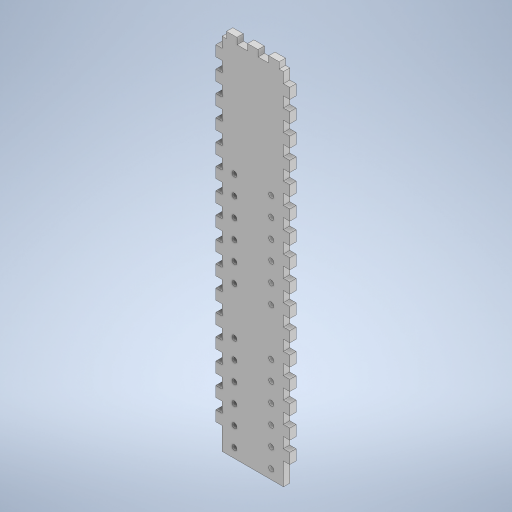
# Autodesk Inventor part: Module_supportX_MFC
Saved by Autodesk Inventor 2023 (Build 270158000, 158)
## iProperties
Created: 2022-11-01
Part Number: Module_supportX_MFC
Material: Generic
Document SubType Name: Modeling
Designer: incep
Density: 1 g/cm^3
Appearance: Default
Author: incep
Autodesk Inventor part; units mm, degrees
ref_plane "YZ Plane" through (0, 0, 0) normal (1, 0, 0) x (0, 1, 0)
ref_plane "XZ Plane" through (0, 0, 0) normal (0, 1, 0) x (-1, 0, 0)
ref_plane "XY Plane" through (0, 0, 0) normal (0, 0, 1) x (1, 0, 0)
sketch "Sketch1" plane through (0, 0, 0) normal (0, 0, 1) x (1, 0, 0)
  line L0 (29.075, 0) -> (29.075, -341.3) construction
  line L1 (29.075, -341.3) -> (-29.075, -341.3)
  line L2 (-29.075, -341.3) -> (-29.075, 0) construction
  line L3 (-5, 6) -> (5, 6)
  line L4 (5, 6) -> (5, 0)
  line L5 (-5, 0) -> (-5, 6)
  line L6 (-29.075, 0) -> (-5, 0) construction
  line L7 (5, 0) -> (29.075, 0) construction
  line L8 (15, 6) -> (25, 6)
  line L9 (25, 6) -> (25, 0)
  line L10 (15, 0) -> (15, 6)
  line L11 (-25, 6) -> (-15, 6)
  line L12 (-15, 6) -> (-15, 0)
  line L13 (-25, 0) -> (-25, 6)
  line L14 (-5, 6) -> (5, 6)
  line L15 (5, 6) -> (5, 0)
  line L16 (-5, 0) -> (-5, 6)
  line L17 (-29.075, 0) -> (-25, 0)
  line L18 (-15, 0) -> (-5, 0)
  line L19 (5, 0) -> (15, 0)
  line L20 (25, 0) -> (29.075, 0)
  line L21 (-35.075, -10) -> (-29.075, -10)
  line L22 (-29.075, -10) -> (-29.075, -20) construction
  line L23 (-29.075, -20) -> (-35.075, -20)
  line L24 (-35.075, -20) -> (-35.075, -10)
  line L25 (-29.075, -20) -> (-29.075, -30)
  line L26 (-29.075, 0) -> (-29.075, -10)
  line L27 (-35.075, -30) -> (-29.075, -30)
  line L28 (-29.075, -40) -> (-29.075, -50)
  line L29 (-29.075, -40) -> (-35.075, -40)
  line L30 (-35.075, -40) -> (-35.075, -30)
  line L31 (-35.075, -50) -> (-29.075, -50)
  line L32 (-29.075, -60) -> (-29.075, -70)
  line L33 (-29.075, -60) -> (-35.075, -60)
  line L34 (-35.075, -60) -> (-35.075, -50)
  line L35 (-35.075, -70) -> (-29.075, -70)
  line L36 (-29.075, -80) -> (-29.075, -90)
  line L37 (-29.075, -80) -> (-35.075, -80)
  line L38 (-35.075, -80) -> (-35.075, -70)
  line L39 (-35.075, -90) -> (-29.075, -90)
  line L40 (-29.075, -100) -> (-29.075, -110)
  line L41 (-29.075, -100) -> (-35.075, -100)
  line L42 (-35.075, -100) -> (-35.075, -90)
  line L43 (-35.075, -110) -> (-29.075, -110)
  line L44 (-29.075, -120) -> (-29.075, -130)
  line L45 (-29.075, -120) -> (-35.075, -120)
  line L46 (-35.075, -120) -> (-35.075, -110)
  line L47 (-35.075, -130) -> (-29.075, -130)
  line L48 (-29.075, -140) -> (-29.075, -150)
  line L49 (-29.075, -140) -> (-35.075, -140)
  line L50 (-35.075, -140) -> (-35.075, -130)
  line L51 (-35.075, -150) -> (-29.075, -150)
  line L52 (-29.075, -160) -> (-29.075, -170)
  line L53 (-29.075, -160) -> (-35.075, -160)
  line L54 (-35.075, -160) -> (-35.075, -150)
  line L55 (-35.075, -170) -> (-29.075, -170)
  line L56 (-29.075, -180) -> (-29.075, -190)
  line L57 (-29.075, -180) -> (-35.075, -180)
  line L58 (-35.075, -180) -> (-35.075, -170)
  line L59 (-35.075, -190) -> (-29.075, -190)
  line L60 (-29.075, -200) -> (-29.075, -210)
  line L61 (-29.075, -200) -> (-35.075, -200)
  line L62 (-35.075, -200) -> (-35.075, -190)
  line L63 (-35.075, -210) -> (-29.075, -210)
  line L64 (-29.075, -220) -> (-29.075, -230)
  line L65 (-29.075, -220) -> (-35.075, -220)
  line L66 (-35.075, -220) -> (-35.075, -210)
  line L67 (-35.075, -230) -> (-29.075, -230)
  line L68 (-29.075, -240) -> (-29.075, -250)
  line L69 (-29.075, -240) -> (-35.075, -240)
  line L70 (-35.075, -240) -> (-35.075, -230)
  line L71 (-35.075, -250) -> (-29.075, -250)
  line L72 (-29.075, -260) -> (-29.075, -270)
  line L73 (-29.075, -260) -> (-35.075, -260)
  line L74 (-35.075, -260) -> (-35.075, -250)
  line L75 (-35.075, -270) -> (-29.075, -270)
  line L76 (-29.075, -280) -> (-29.075, -290)
  line L77 (-29.075, -280) -> (-35.075, -280)
  line L78 (-35.075, -280) -> (-35.075, -270)
  line L79 (-35.075, -290) -> (-29.075, -290)
  line L80 (-29.075, -300) -> (-29.075, -310)
  line L81 (-29.075, -300) -> (-35.075, -300)
  line L82 (-35.075, -300) -> (-35.075, -290)
  line L83 (-35.075, -310) -> (-29.075, -310)
  line L84 (-29.075, -320) -> (-29.075, -330)
  line L85 (-29.075, -320) -> (-35.075, -320)
  line L86 (-35.075, -320) -> (-35.075, -310)
  line L87 (-29.075, -330) -> (-29.075, -341.3)
  line L88 (0, 0) -> (0, -341.3) construction
  line L89 (29.075, -341.3) -> (29.075, 0) construction
  line L90 (35.075, -10) -> (29.075, -10)
  line L91 (29.075, -10) -> (29.075, -20) construction
  line L92 (29.075, -20) -> (35.075, -20)
  line L93 (35.075, -20) -> (35.075, -10)
  line L94 (29.075, -20) -> (29.075, -30)
  line L95 (29.075, 0) -> (29.075, -10)
  line L96 (35.075, -30) -> (29.075, -30)
  line L97 (29.075, -40) -> (29.075, -50)
  line L98 (29.075, -40) -> (35.075, -40)
  line L99 (35.075, -40) -> (35.075, -30)
  line L100 (35.075, -50) -> (29.075, -50)
  line L101 (29.075, -60) -> (29.075, -70)
  line L102 (29.075, -60) -> (35.075, -60)
  line L103 (35.075, -60) -> (35.075, -50)
  line L104 (35.075, -70) -> (29.075, -70)
  line L105 (29.075, -80) -> (29.075, -90)
  line L106 (29.075, -80) -> (35.075, -80)
  line L107 (35.075, -80) -> (35.075, -70)
  line L108 (35.075, -90) -> (29.075, -90)
  line L109 (29.075, -100) -> (29.075, -110)
  line L110 (29.075, -100) -> (35.075, -100)
  line L111 (35.075, -100) -> (35.075, -90)
  line L112 (35.075, -110) -> (29.075, -110)
  line L113 (29.075, -120) -> (29.075, -130)
  line L114 (29.075, -120) -> (35.075, -120)
  line L115 (35.075, -120) -> (35.075, -110)
  line L116 (35.075, -130) -> (29.075, -130)
  line L117 (29.075, -140) -> (29.075, -150)
  line L118 (29.075, -140) -> (35.075, -140)
  line L119 (35.075, -140) -> (35.075, -130)
  line L120 (35.075, -150) -> (29.075, -150)
  line L121 (29.075, -160) -> (29.075, -170)
  line L122 (29.075, -160) -> (35.075, -160)
  line L123 (35.075, -160) -> (35.075, -150)
  line L124 (35.075, -170) -> (29.075, -170)
  line L125 (29.075, -180) -> (29.075, -190)
  line L126 (29.075, -180) -> (35.075, -180)
  line L127 (35.075, -180) -> (35.075, -170)
  line L128 (35.075, -190) -> (29.075, -190)
  line L129 (29.075, -200) -> (29.075, -210)
  line L130 (29.075, -200) -> (35.075, -200)
  line L131 (35.075, -200) -> (35.075, -190)
  line L132 (35.075, -210) -> (29.075, -210)
  line L133 (29.075, -220) -> (29.075, -230)
  line L134 (29.075, -220) -> (35.075, -220)
  line L135 (35.075, -220) -> (35.075, -210)
  line L136 (35.075, -230) -> (29.075, -230)
  line L137 (29.075, -240) -> (29.075, -250)
  line L138 (29.075, -240) -> (35.075, -240)
  line L139 (35.075, -240) -> (35.075, -230)
  line L140 (35.075, -250) -> (29.075, -250)
  line L141 (29.075, -260) -> (29.075, -270)
  line L142 (29.075, -260) -> (35.075, -260)
  line L143 (35.075, -260) -> (35.075, -250)
  line L144 (35.075, -270) -> (29.075, -270)
  line L145 (29.075, -280) -> (29.075, -290)
  line L146 (29.075, -280) -> (35.075, -280)
  line L147 (35.075, -280) -> (35.075, -270)
  line L148 (35.075, -290) -> (29.075, -290)
  line L149 (29.075, -300) -> (29.075, -310)
  line L150 (29.075, -300) -> (35.075, -300)
  line L151 (35.075, -300) -> (35.075, -290)
  line L152 (35.075, -310) -> (29.075, -310)
  line L153 (29.075, -320) -> (29.075, -330)
  line L154 (29.075, -320) -> (35.075, -320)
  line L155 (35.075, -320) -> (35.075, -310)
  line L156 (29.075, -330) -> (29.075, -341.3)
  circle A0 centre (17.5, -332.3) radius 2.4
  circle A1 centre (17.5, -197.5) radius 2.4
  circle A2 centre (17.5, -314.3) radius 2.4
  circle A3 centre (17.5, -179.5) radius 2.4
  circle A4 centre (17.5, -296.3) radius 2.4
  circle A5 centre (17.5, -161.5) radius 2.4
  circle A6 centre (17.5, -278.3) radius 2.4
  circle A7 centre (17.5, -143.5) radius 2.4
  circle A8 centre (17.5, -260.3) radius 2.4
  circle A9 centre (17.5, -125.5) radius 2.4
  circle A10 centre (17.5, -242.3) radius 2.4
  circle A11 centre (17.5, -107.5) radius 2.4
  circle A12 centre (-17.5, -332.3) radius 2.4
  circle A13 centre (-17.5, -197.5) radius 2.4
  circle A14 centre (-17.5, -314.3) radius 2.4
  circle A15 centre (-17.5, -179.5) radius 2.4
  circle A16 centre (-17.5, -296.3) radius 2.4
  circle A17 centre (-17.5, -161.5) radius 2.4
  circle A18 centre (-17.5, -278.3) radius 2.4
  circle A19 centre (-17.5, -143.5) radius 2.4
  circle A20 centre (-17.5, -260.3) radius 2.4
  circle A21 centre (-17.5, -125.5) radius 2.4
  circle A22 centre (-17.5, -242.3) radius 2.4
  circle A23 centre (-17.5, -107.5) radius 2.4
  point P0 (0, 6)
  point P1 (20, 0)
  point P2 (20, 0)
  point P3 (20, 6)
  point P4 (-20, 0)
  point P5 (-20, 0)
  point P6 (-20, 6)
  point P7 (0, 6)
  point P8 (10, 0)
  dimension "d7" = 341.3
  dimension "d9" = 58.15
  dimension "d11" = 10
  dimension "d12" = 6
  dimension "d38" = 20
  dimension "d49" = 20
  dimension "d58" = 6
  dimension "d60" = 10
  dimension "d61" = 10
  dimension "d62" = 10
  dimension "d69" = 20
  dimension "d75" = 4.8
  dimension "d76" = 17.5
  dimension "d77" = 9
  dimension "d78" = 4.8
  dimension "d80" = 134.8
  dimension "d83" = 18
  dimension "d86" = 35
  constraints: 314 end point, 80 symmetric about line, 24 centre point, 7 horizontal, 6 parallel, 5 vertical, 4 collinear, 4 perpendicular, 3 midpoint, 3 vertical alignment, 2 coincident, 1 horizontal alignment, 209 other
  measures "d7" distance of L1.end L2.end
  measures "d9" distance of L0.end L1.end
  measures "d11" distance of L3.start L3.end
  measures "d12" distance of L5.start L3.start
  measures "d38" distance of point (0, 0) point (20, 0)
  measures "d49" distance of point (0, 0) point (-20, 0)
  measures "d58" distance between parallel lines of L22 L24
  measures "d60" distance between parallel lines of L23 L21
  measures "d61" distance of L22.end L25.end
  measures "d62" distance from line of L21 point (0, 0)
  measures "d69" distance of L22.end L28.start
  measures "d75" diameter of A0
  measures "d76" horizontal distance of L88.end A0.centre
  measures "d77" vertical distance of A0.centre L88.end
  measures "d78" diameter of A1
  measures "d80" distance of A0.centre A1.centre
  measures "d83" distance of A0.centre A2.centre
  measures "d86" distance of A0.centre A12.centre
extrude "Extrusion1" add sketch "Sketch1" along normal blind 6
equation "\"d7\" = supportL"
equation "\"d9\" = supportXW"
equation "\"d11\" = fingerW"
equation "\"d12\" = fingerH"
equation "\"d38\" = fingerSpacing"
equation "\"d49\" = fingerSpacing"
equation "\"d58\" = fingerH"
equation "\"d60\" = fingerW"
equation "\"d61\" = fingerSpacing - fingerW"
equation "\"d62\" = 0.5 * fingerSpacing"
equation "\"d69\" = fingerSpacing"
equation "\"d75\" = clearanceM4"
equation "\"d76\" = 0.5 * actuatorMountX"
equation "\"d77\" = 0.5 * actuatorMountY"
equation "\"d78\" = d79"
equation "\"d80\" = acutatorMountSpacing"
equation "\"d83\" = actuatorMountY"
equation "\"d86\" = actuatorMountX"
equation "\"d54\" = thickness"
equation "\"moduleWidth\" = 118"
equation "\"moduleHeight\" = 96"
equation "\"moduleMountD\" = 6.8"
equation "\"moduleCornerR\" = 5"
equation "\"d4\" = moduleCornerR"
equation "\"d5\" = moduleMountD"
equation "\"d6\" = moduleMountD"
equation "\"d8\" = moduleMountD"
equation "\"d10\" = moduleMountD"
equation "\"moduleOpeningR\" = 25"
equation "\"d13\" = moduleOpeningR"
equation "\"thickness\" = 6"
equation "\"d15\" = thickness"
equation "\"d16\" = 0"
equation "\"kerf\" = 0.15"
equation "\"fingerW\" = 10"
equation "\"fingerSpacing\" = 20"
equation "\"fingerholeW\" = fingerW - 2 * kerf"
equation "\"fingerholeH\" = thickness - kerf"
equation "\"moduleMountClearance\" = 19"
equation "\"actuatorW\" = 28"
equation "\"actuatorH\" = 40.8"
equation "\"openingMFC\" = 45"
equation "\"d28\" = thickness"
equation "\"d29\" = thickness"
equation "\"d30\" = 0.5 * actuatorH + thickness"
equation "\"d32\" = fingerholeH"
equation "\"d33\" = fingerholeW"
equation "\"d41\" = fingerholeH"
equation "\"d42\" = fingerholeW"
equation "\"supportSpacingFromMounting\" = 15"
equation "\"d52\" = 58.075"
equation "\"d53\" = 9.475"
equation "\"d0\" = moduleHeight"
equation "\"d1\" = moduleWidth"
equation "\"d17\" = openingMFC"
equation "\"d19\" = moduleMountClearance"
equation "\"d31\" = supportSpacingFromMounting"
equation "\"supportXW\" = -2 * thickness + moduleMountW - 2 * supportSpacingFromMounting + kerf"
equation "\"chairThickness\" = 12.7"
equation "\"supportL\" = -chairThickness + dildoL + actuatorMountL - thickness"
equation "\"fingerH\" = thickness"
equation "\"d18\" = fingerH"
equation "\"d24\" = supportL"
equation "\"d44\" = thickness"
equation "\"d47\" = 0"
equation "\"d64\" = 9.4"
equation "\"supportsCTCZ\" = d64"
equation "\"clearanceM4\" = 4.8"
equation "\"actuatorMountX\" = 35"
equation "\"actuatorMountY\" = 18"
equation "\"acutatorMountSpacing\" = 134.8"
equation "\"d79\" = 4.8"
equation "\"moduleMountW\" = 100"
equation "\"dildoL\" = 170"
equation "\"actuatorMountL\" = 190"
body "Solid1"
